# Autodesk Inventor part: ANSI L 3 x 2 x 1_4 00000011
Saved by Autodesk Inventor 2021 (Build 250183000, 183)
## iProperties
Created: 2007-11-22
Part Number: ANSI L 3 x 2 x 1_4 00000011
Material: Generic
Document SubType Name: Modeling
Standard: ANSI
Designer: nino.caldarola
Size Designation: L 3 x 2 x 1/4
Stock Number: L 3 x 2 x 1/4
Density: 1 g/cm^3
Appearance: Default
_FrameMemberDoc: Frame Member File
_Version: 12.0.0
_CCFamilyMember: 6
_CCFamilyDisplayName: ANSI L (Unequal angles) - Angle Steel
G_L: 33.250 in
G_W: 2.000 in
G_H: 3.000 in
Author: nino.caldarola
Autodesk Inventor part; units mm, degrees
ref_plane "YZ Plane" through (0, 0, 0) normal (1, 0, 0) x (0, 1, 0)
ref_plane "Start plane" through (0, 0, 0) normal (0, 0, 1) x (1, 0, 0)
ref_plane "End plane" through (0, 0, 844.55) normal (0, 0, 1) x (1, 0, 0)
sketch "Sketch" plane through (0, 0, 0) normal (0, 0, 1) x (1, 0, 0)
  line L0 (0, 76.2) -> (0, 0)
  line L1 (0, 0) -> (50.8, 0)
  line L2 (50.8, 0) -> (50.8, 4.35)
  line L3 (48.8, 6.35) -> (14.224, 6.35)
  line L4 (6.35, 14.224) -> (6.35, 74.2)
  line L5 (4.35, 76.2) -> (0, 76.2)
  line L6 (-7.0414, 0) -> (21.5385, 0) construction
  line L7 (0, -8.0414) -> (0, 34.5385) construction
  arc A0 (6.35, 14.224) -> (14.224, 6.35) centre (14.224, 14.224) ccw
  arc A1 (50.8, 4.35) -> (48.8, 6.35) centre (48.8, 4.35) ccw
  arc A2 (6.35, 74.2) -> (4.35, 76.2) centre (4.35, 74.2) ccw
  line L8 (0, 93.5453) -> (0, -24.9725) construction
  line L9 (-18.6925, 0) -> (62.8653, 0) construction
  point P0 (50.8, 6.35)
  point P1 (6.35, 6.35)
  point P2 (6.35, 76.2)
  dimension "d12" = 6.35
  dimension "d13" = 76.2
  dimension "d14" = 50.8
  dimension "d15" = 0
  dimension "d16" = 6.35
  dimension "d17" = 0
  dimension "d18" = 7.874
  dimension "d19" = 2
  constraints: 16 end point, 6 point on circle, 6 point on line, 6 tangent, 3 centre point, 2 collinear, 2 parallel, 1 equal radius
  measures "d12" distance between parallel lines of L4 L0
  measures "d13" distance of L0.start L1.start
  measures "d14" distance of L1.start L1.end
  measures "d15" distance between parallel lines of L6 L1
  measures "d16" distance between parallel lines of L1 L3
  measures "d17" distance between parallel lines of L7 L0
  measures "d18" radius of A0
  measures "d19" radius of A1
extrude "Body" add sketch "Sketch" along normal up to surface (844.55 mm away) from surface at 0
sketch "Sketch3" plane through (6.35, 14.224, 844.55) normal (1, 0, 0) x (0, 0, -1)
  line L0 (0, 59.976) -> (0, 0) projected
  line L1 (844.55, 59.976) -> (844.55, 0) projected
  line L2 (844.55, 59.976) -> (0, 59.976) projected
  line L3 (0, 36.576) -> (844.55, 36.576) construction
  line L4 (844.55, 61.976) -> (0, 61.976) projected
  point P0 (76.2, 36.576)
  point P1 (422.275, 36.576)
  point P2 (768.35, 36.576)
  dimension "d22" = 76.2
  dimension "d23" = 422.275
  dimension "d24" = 768.35
  dimension "d32" = 25.4
  constraints: 4 point on line, 2 end point, 1 midpoint, 1 parallel
  measures "d22" distance from line of L0 point (76.2, 36.576)
  measures "d23" distance from line of point (422.275, 36.576) L0
  measures "d24" distance from line of point (768.35, 36.576) L0
  measures "d32" distance between parallel lines of L4 L3
hole "Hole1" at (6.35, 50.8, 768.35) at (6.35, 50.8, 422.275) at (6.35, 50.8, 76.2) direction (-1, 0, 0) diameter 15.875 end through all
equation "\"d12\" = G_T"
equation "\"d13\" = G_H"
equation "\"d14\" = G_W"
equation "\"d16\" = G_T"
equation "\"d18\" = G_IR"
equation "\"d4\" = G_L"
equation "\"G_W\" = 50.8"
equation "\"G_H\" = 76.2"
equation "\"G_T\" = 6.35"
equation "\"G_ER\" = 4.064"
equation "\"G_IR\" = 7.874"
equation "\"G_L\" = B_L + G_OFFSET_START + G_OFFSET_END"
equation "\"ex\" = 0"
equation "\"ey\" = 0"
equation "\"G_OFFSET_START\" = 0"
equation "\"G_OFFSET_END\" = 0"
equation "\"d21\" = G_OFFSET_END + B_L"
equation "\"B_L\" = 844.55"
body "Solid1"
